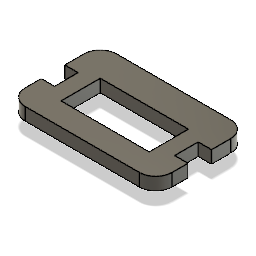
SF2_Cap_Jan_7_2019 v5 (Autodesk Fusion 360 design; units mm, degrees)
Autodesk Fusion 360 part; units mm, degrees
note: some values were not read from the file. Set by a fixed rule: which sketch regions a step uses.
sketch "Sketch1" plane through (0, 0, 0) normal (0, 1, 0) x (1, 0, 0)
  line L0 (-9, 0) -> (0, 0)
  line L1 (-36, 0) -> (-45, 0)
  line L2 (-36, 28) -> (-45, 28)
  line L3 (-36, 0) -> (-9, 0)
  line L4 (-34.15, 28) -> (-34.15, 24)
  line L5 (-9, 28) -> (-10, 28)
  line L6 (-45, 28) -> (-45, 0)
  line L7 (0, 28) -> (0, 0)
  line L8 (-34.15, 28) -> (-36, 28)
  line L9 (-34.15, 28) -> (-10, 28)
  line L10 (-34.15, 24) -> (-10, 24)
  line L11 (-45, 0) -> (-36, 0)
  line L12 (0, 28) -> (-9, 28)
  line L13 (-36, 7) -> (-9, 7)
  line L14 (-9, 7) -> (-9, 19)
  line L15 (-9, 19) -> (-36, 19)
  line L16 (-36, 19) -> (-36, 7)
  line L17 (-40.9, 17.1) -> (-40.9, 9.9)
  line L18 (-40.9, 9.9) -> (-45, 9.9)
  line L19 (-40.9, 17.1) -> (-45, 17.1)
  line L20 (-4.1, 17.1) -> (-4.1, 9.9)
  line L21 (-4.1, 17.1) -> (0, 17.1)
  line L22 (-4.1, 9.9) -> (0, 9.9)
  line L23 (0, 28) -> (-9.5, 28)
  line L24 (-9.5, 28) -> (-9.5, 24)
  line L25 (-10, 24) -> (-9.5, 24)
  point P0 (-45, 0)
  dimension "d171" = 9
  dimension "d238" = 9.5
  constraint coincident L0.end L7.end
  constraint parallel L0 L3
  constraint coincident P0 L1.end
  constraint perpendicular L1 L6
  constraint perpendicular L0 L7
  constraint vertical L4
  constraint perpendicular L4 L8
  constraint perpendicular L7 L12
  constraint horizontal L13
  constraint vertical L14
  constraint horizontal L15
  constraint vertical L16
  constraint coincident L6 L18.end
  constraint perpendicular L6 L18
  constraint coincident L6 L19.end
  constraint perpendicular L6 L19
  constraint coincident L7 L21.end
  constraint perpendicular L7 L21
  constraint coincident L7 L22.end
  constraint perpendicular L7 L22
  constraint perpendicular L7 L23
  constraint perpendicular L24 L25
  measures "d171" distance of L5.start L14.end
  measures "d238" distance of L7.start L23.end
extrude "Extrude78" add sketch "Sketch1" against normal blind 4 contours L4 L5 L9 L10 L24 L25 makes body 1
extrude "Extrude76" add sketch "Sketch1" along normal blind 3.9 separate body contours L0 L1 L2 L3 L4 L5 L6 L7 L8 L10 L11 L12 L17 L18 L19 L20 L21 L22 L23 L24 L25 | L4 L5 L9 L10 L24 L25 makes body 2
extrude "Extrude77" add sketch "Sketch1" along normal blind 3.5 contours L4 L5 L9 L10 L24 L25 bodies 2
fillet "Fillet20" radius 5 4 edges at (-45, 1.95, 0) (0, 1.95, 0) (0, 1.95, -28) (-45, 1.95, -28) on bodies 2
move_face "OffsetFaces2" offset -0.1 1 faces at (-9.5, -1.3333, -26.6667) on bodies 1
